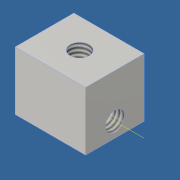
# Autodesk Inventor part: Alu_Belt_tens_3
Saved by Autodesk Inventor 2016 (Build 200138000, 138)
## iProperties
Created: 2016-03-08
Part Number: Alu_Belt_tens_3
Material: Aluminium 6061
Document SubType Name: Modeling
Designer: 4ndreas
Density: 2.7 g/cm^3
Appearance: Aluminium - flach
Mass: 2.8369 g
Surface Area: 8.37376 cm^2
Volume: 1.0507 cm^3
Author: 4ndreas
Autodesk Inventor part; units mm, degrees
note: some values were not read from the file. Chosen so that the rebuilt part matches the saved one: direction of "Bohrung2".
ref_plane "YZ Plane" through (0, 0, 0) normal (1, 0, 0) x (0, 1, 0)
ref_plane "XZ Plane" through (0, 0, 0) normal (0, 1, 0) x (-1, 0, 0)
ref_plane "XY Plane" through (0, 0, 0) normal (0, 0, 1) x (1, 0, 0)
sketch "Skizze1" plane through (0, 0, 0) normal (0, 0, 1) x (1, 0, 0)
  line L0 (0, 0) -> (12, 0)
  line L1 (12, 0) -> (12, 10)
  line L2 (12, 10) -> (0, 10)
  line L3 (0, 10) -> (0, 0)
  dimension "d0" = 10
  dimension "d1" = 12
  constraints: 8 end point, 2 parallel, 1 horizontal, 1 perpendicular
  measures "d0" distance between parallel lines of L0 L2
  measures "d1" distance between parallel lines of L1 L3
extrude "Extrusion1" add sketch "Skizze1" along normal blind 10
sketch "Skizze2" plane through (12, 0, 0) normal (1, 0, 0) x (0, 0, -1)
  line L0 (0, 0) -> (0, 10) projected
  line L1 (0, 10) -> (-10, 10) projected
  line L2 (-10, 0) -> (-10, 10) projected
  line L3 (0, 0) -> (-10, 0) projected
  line L4 (-10, 5) -> (0, 5) construction
  point P0 (-2.5, 5)
  dimension "d4" = 2.5
  constraints: 2 end point, 2 midpoint, 1 point on line
  measures "d4" distance from line of point (-2.5, 5) L0
hole "Bohrung1" at (12, 5, 2.5) direction (-1, 0, 0) diameter 3.242 depth 11.8 tip angle 118 thread size "M4x0.7" class "6H" standard "ISO Metric profile"
sketch "Skizze3" plane through (0, 0, 10) normal (0, 0, 1) x (1, 0, 0)
  line L0 (0, 0) -> (12, 0) projected
  line L1 (12, 0) -> (12, 10) projected
  line L2 (12, 10) -> (0, 10) projected
  line L3 (0, 10) -> (0, 0) projected
  line L4 (12, 6.621) -> (12, 3.379) projected
  line L5 (0.2, 3.379) -> (0.2, 6.621) projected
  line L6 (-2.4, 5) -> (14.4, 5) projected
  line L7 (6, 0) -> (6, 10) construction
  point P0 (6, 5)
  point P1 (6, 5)
  constraints: 5 midpoint, 2 end point
hole "Bohrung2" at (6, 5, 10) direction (0, 0, -1) diameter 3.242 end up to surface thread size "M4x0.7" class "6H" standard "ISO Metric profile"
